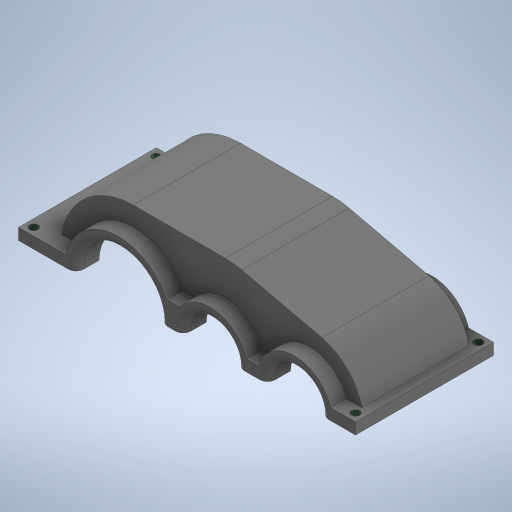
# Autodesk Inventor part: Part9
Saved by Autodesk Inventor 2023.2 (Build 272271030, 271C)
## iProperties
Created: 2023-01-29
Part Number: Part9
Material: Generic
Document SubType Name: Modeling
Designer: Merve Babacan
Density: 1 g/cm^3
Appearance: Green Polished
Author: Merve Babacan
Autodesk Inventor part; units mm, degrees
ref_plane "YZ Plane" through (0, 0, 0) normal (1, 0, 0) x (0, 1, 0)
ref_plane "XZ Plane" through (0, 0, 0) normal (0, 1, 0) x (-1, 0, 0)
sketch "Sketch1" plane through (0, 0, 0) normal (0, 0, 1) x (1, 0, 0)
  arc A0 (44.2099, 260.8514) -> (-65.7901, 260.8514) centre (-10.7901, 260.8514) ccw
  arc A1 (52.4554, 290.8514) -> (-79.1641, 275.8514) centre (-10.7901, 260.8514) ccw
  arc A2 (144.2099, 260.8514) -> (74.2099, 260.8514) centre (109.2099, 260.8514) ccw
  arc A3 (156.9068, 275.8514) -> (69.2099, 290.8514) centre (109.2099, 260.8514) ccw
  arc A4 (254.2099, 260.8514) -> (184.2099, 260.8514) centre (219.2099, 260.8514) ccw
  arc A5 (266.9068, 275.8514) -> (171.5129, 275.8514) centre (219.2099, 260.8514) ccw
  line L0 (-140.7901, 260.8514) -> (-140.7901, 275.8514)
  line L1 (299.2099, 275.8514) -> (299.2099, 260.8514)
  line L2 (-140.7901, 275.8514) -> (-79.1641, 275.8514)
  line L3 (-140.7901, 260.8514) -> (-65.7901, 260.8514)
  line L4 (52.4554, 290.8514) -> (69.2099, 290.8514)
  line L5 (44.2099, 260.8514) -> (74.2099, 260.8514)
  line L6 (156.9068, 275.8514) -> (171.5129, 275.8514)
  line L7 (266.9068, 275.8514) -> (299.2099, 275.8514)
  line L8 (144.2099, 260.8514) -> (184.2099, 260.8514)
  line L9 (254.2099, 260.8514) -> (299.2099, 260.8514)
  arc A6 (81.7099, 282.502) -> (-104.5984, 275.8514) centre (-10.7901, 260.8514) ccw
  circle A7 centre (306.7595, 253.9492) radius 1.6696
  arc A8 (287.5838, 275.8514) -> (235.119, 329.0196) centre (219.2099, 260.8514) ccw
  line L10 (-10.7901, 355.8514) -> (109.2099, 355.8514)
  line L11 (130.8008, 353.3653) -> (235.119, 329.0196)
  arc A9 (199.6644, 289.8854) -> (193.869, 303.954) centre (109.2099, 260.8514) ccw
  arc A10 (130.8008, 353.3653) -> (109.2099, 355.8514) centre (109.2099, 260.8514) ccw
  point P0 (0, 0)
  dimension "d0" = 110
  dimension "d1" = 140
  dimension "d2" = 70
  dimension "d3" = 100
  dimension "d4" = 70
  dimension "d5" = 100
  dimension "d6" = 120
  dimension "d7" = 110
  dimension "d8" = 130
  dimension "d9" = 440
  dimension "d10" = 15
  dimension "d12" = 190
  dimension "d14" = 140
  constraints: 24 end point, 24 point on circle, 11 centre point, 6 coincident, 5 horizontal, 3 perpendicular, 3 tangent, 2 point on line, 1 vertical
  measures "d0" diameter of A0
  measures "d1" diameter of A1
  measures "d2" diameter of A2
  measures "d3" diameter of A3
  measures "d4" diameter of A4
  measures "d5" diameter of A5
  measures "d6" distance of A2.centre A0.centre
  measures "d7" distance of A4.centre A2.centre
  measures "d8" distance of A0.centre L0.start
  measures "d9" distance of L0.start L1.end
  measures "d10" distance of L0.start L0.end
  measures "d12" diameter of A6
  measures "d14" diameter of A8
extrude "Extrusion1" add sketch "Sketch1" along normal blind 30 contours A0 L3 L0 L2 A1 L4 A3 A6 A2 L5 | A6 A3 L6 A5 A9 A4 L8 A2 | A9 A5 L7 L1 L9 A4
extrude "Extrusion2" add sketch "Sketch1" along normal blind 10 contours A6 L10 A10 L11 A8 L7 A5 L6 A3 | A3 L4 A1 L2 A6
sketch "Sketch2" plane through (0, 0, 0) normal (0, 0, -1) x (-1, 0, 0)
  arc A0 (-235.119, 329.0196) -> (-287.5838, 275.8514) centre (-219.2099, 260.8514) ccw projected
  line L0 (-235.119, 329.0196) -> (-130.8008, 353.3653) projected
  line L1 (-109.2099, 355.8514) -> (10.7901, 355.8514) projected
  arc A1 (-109.2099, 355.8514) -> (-130.8008, 353.3653) centre (-109.2099, 260.8514) ccw projected
  arc A2 (104.5984, 275.8514) -> (10.7901, 355.8514) centre (10.7901, 260.8514) ccw projected
  arc A3 (94.4561, 275.8514) -> (10.7901, 345.8514) centre (10.7901, 260.8514) ccw
  line L2 (10.7901, 345.8514) -> (-109.2099, 345.8514)
  arc A4 (-109.2099, 345.8514) -> (-128.528, 343.627) centre (-109.2099, 260.8514) ccw
  line L3 (-128.528, 343.627) -> (-232.8462, 319.2812)
  arc A5 (-232.8462, 319.2812) -> (-277.8161, 273.7085) centre (-219.2099, 260.8514) ccw
  arc A6 (104.5984, 275.8514) -> (10.7901, 355.8514) centre (10.7901, 260.8514) ccw projected
  line L4 (-287.5838, 275.8514) -> (-277.3046, 275.8514)
  line L5 (94.4561, 275.8514) -> (104.5984, 275.8514)
  point P0 (0, 0)
  dimension "d19" = 10
  constraints: 8 end point, 7 point on circle, 3 centre point, 3 other
  measures "d19" distance between parallel lines of L0 L3
extrude "Extrusion3" add sketch "Sketch2" along normal blind 130
ref_plane "Work Plane1" through (0, 0, -60) normal (0, 0, -1) x (-1, 0, 0)
mirror "Mirror1" about plane through (0, 0, -60) normal (0, 0, -1) of "Extrusion1", "Extrusion2"
sketch "Sketch3" plane through (0, 0, -60) normal (0, 0, -1) x (-1, 0, 0)
  line L0 (-299.2099, 260.8514) -> (-299.2099, 275.8514) projected
  line L1 (-277.3046, 275.8514) -> (-299.2099, 275.8514)
  line L2 (-299.2099, 275.8514) -> (-299.2099, 260.8514)
  line L3 (-299.2099, 260.8514) -> (-277.3046, 260.8514)
  line L4 (-277.3046, 260.8514) -> (-277.3046, 275.8514)
  line L5 (140.7901, 275.8514) -> (140.7901, 260.8514) projected
  line L6 (94.4561, 275.8514) -> (140.7901, 275.8514)
  line L7 (140.7901, 275.8514) -> (140.7901, 260.8514)
  line L8 (140.7901, 260.8514) -> (94.4561, 260.8514)
  line L9 (94.4561, 260.8514) -> (94.4561, 275.8514)
  point P0 (0, 0)
  constraints: 16 end point, 4 parallel, 2 horizontal, 2 perpendicular
extrude "Extrusion4" add sketch "Sketch3" along normal through all both and the other way through all
fillet "Fillet1" radius 10 6 edges at (-10.7901, 315.8514, 30) (109.2099, 295.8514, 30) (219.2099, 295.8514, 30) (219.2099, 295.8514, -150) (109.2099, 295.8514, -150) (-10.7901, 315.8514, -150)
sketch "Sketch4" plane through (-140.7901, 275.8514, 30) normal (0, 1, 0) x (1, 0, 0)
  point P0 (10, 10)
hole "Hole1" at (-130.7901, 275.8514, 20) direction (0, -1, 0) diameter 11 end through all
sketch "Sketch5" plane through (-140.7901, 275.8514, 30) normal (0, 1, 0) x (1, 0, 0)
  point P0 (10, 170)
hole "Hole2" at (-130.7901, 275.8514, -140) direction (0, -1, 0) diameter 11 end through all
sketch "Sketch6" plane through (266.9068, 275.8514, 30) normal (0, 1, 0) x (1, 0, 0)
  point P0 (22.303, 10)
hole "Hole3" at (289.2099, 275.8514, 20) direction (0, -1, 0) diameter 11 end through all
sketch "Sketch7" plane through (266.9068, 275.8514, 30) normal (0, 1, 0) x (1, 0, 0)
  point P0 (22.303, 170)
hole "Hole4" at (289.2099, 275.8514, -140) direction (0, -1, 0) diameter 11 end through all
body "Solid1"
